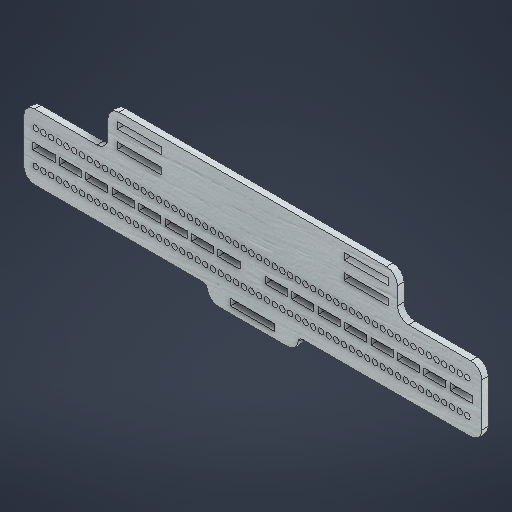
# Autodesk Inventor part: side_frame
Saved by Autodesk Inventor 2025.3 (Build 293356030, 356C)
## iProperties
Created: 2025-09-04
Part Number: side_frame
Material: 木材 (楓木)
Document SubType Name: Modeling
Designer: 陳泓任
Density: 0.67 g/cm^3
Appearance: 木材 - 白色刷漆
Author: 陳泓任
Autodesk Inventor part; units mm, degrees
ref_plane "YZ Plane" through (0, 0, 0) normal (1, 0, 0) x (0, 1, 0)
ref_plane "XZ Plane" through (0, 0, 0) normal (0, 1, 0) x (-1, 0, 0)
ref_plane "XY Plane" through (0, 0, 0) normal (0, 0, 1) x (1, 0, 0)
sketch "草圖1" plane through (0, 0, 0) normal (0, 0, 1) x (1, 0, 0)
  line L0 (41.49, 17.7685) -> (41.49, 20.7685)
  line L1 (41.49, 20.7685) -> (61.49, 20.7685)
  line L2 (61.49, 20.7685) -> (61.49, 17.7685)
  line L3 (61.49, 17.7685) -> (41.49, 17.7685)
  arc A0 (99, -14.8985) -> (104, -9.8985) centre (99, -9.8985) ccw
  arc A1 (-104, -9.8985) -> (-99, -14.8985) centre (-99, -9.8985) ccw
  line L4 (-61.49, 17.7685) -> (-61.49, 20.7685)
  line L5 (-61.49, 20.7685) -> (-41.49, 20.7685)
  line L6 (-41.49, 20.7685) -> (-41.49, 17.7685)
  line L7 (-41.49, 17.7685) -> (-61.49, 17.7685)
  arc A2 (65.74, 27.7685) -> (60.74, 32.7685) centre (60.74, 27.7685) ccw
  circle A3 centre (-98.5092, 7.5) radius 1.25
  circle A4 centre (-98.5092, -7.5) radius 1.25
  arc A5 (-70.74, 14.8985) -> (-65.74, 19.8985) centre (-70.74, 19.8985) ccw
  arc A6 (104, 9.8985) -> (99, 14.8985) centre (99, 9.8985) ccw
  arc A7 (-99, 14.8985) -> (-104, 9.8985) centre (-99, 9.8985) ccw
  arc A8 (65.74, 19.8985) -> (70.74, 14.8985) centre (70.74, 19.8985) ccw
  line L8 (-99, -14.8985) -> (-22.615, -14.8985)
  arc A9 (15.6624, -21.0852) -> (20.6286, -16.6661) centre (15.6624, -16.0852) ccw
  arc A10 (22.615, -14.8985) -> (20.6286, -16.6661) centre (22.615, -16.8985) ccw
  line L9 (-10, -18.0852) -> (-10, -15.0852)
  line L10 (-10, -15.0852) -> (10, -15.0852)
  line L11 (10, -15.0852) -> (10, -18.0852)
  line L12 (10, -18.0852) -> (-10, -18.0852)
  arc A11 (-20.6286, -16.6661) -> (-22.615, -14.8985) centre (-22.615, -16.8985) ccw
  arc A12 (-20.6286, -16.6661) -> (-15.6624, -21.0852) centre (-15.6624, -16.0852) ccw
  line L13 (-65.74, 27.7685) -> (-65.74, 19.8985)
  line L14 (-104, 9.8985) -> (-104, -9.8985)
  line L15 (104, 9.8985) -> (104, -9.8985)
  line L16 (-15.6624, -21.0852) -> (15.6624, -21.0852)
  line L17 (22.615, -14.8985) -> (99, -14.8985)
  line L18 (70.74, 14.8985) -> (99, 14.8985)
  line L19 (-99, 14.8985) -> (-70.74, 14.8985)
  line L20 (0, -35.3826) -> (0, 51.5191)
  line L21 (-104.9871, 0) -> (119.3176, 0)
  circle A13 centre (-95.0092, 7.5) radius 1.25
  circle A14 centre (-95.0092, -7.5) radius 1.25
  circle A15 centre (-91.5092, 7.5) radius 1.25
  circle A16 centre (-91.5092, -7.5) radius 1.25
  circle A17 centre (-88.0092, 7.5) radius 1.25
  circle A18 centre (-88.0092, -7.5) radius 1.25
  circle A19 centre (-84.5092, 7.5) radius 1.25
  circle A20 centre (-84.5092, -7.5) radius 1.25
  circle A21 centre (-81.0092, 7.5) radius 1.25
  circle A22 centre (-81.0092, -7.5) radius 1.25
  circle A23 centre (-77.5092, 7.5) radius 1.25
  circle A24 centre (-77.5092, -7.5) radius 1.25
  circle A25 centre (-74.0092, 7.5) radius 1.25
  circle A26 centre (-74.0092, -7.5) radius 1.25
  circle A27 centre (-70.5092, 7.5) radius 1.25
  circle A28 centre (-70.5092, -7.5) radius 1.25
  circle A29 centre (-67.0092, 7.5) radius 1.25
  circle A30 centre (-67.0092, -7.5) radius 1.25
  circle A31 centre (-63.5092, 7.5) radius 1.25
  circle A32 centre (-63.5092, -7.5) radius 1.25
  circle A33 centre (-60.0092, 7.5) radius 1.25
  circle A34 centre (-60.0092, -7.5) radius 1.25
  circle A35 centre (-56.5092, 7.5) radius 1.25
  circle A36 centre (-56.5092, -7.5) radius 1.25
  circle A37 centre (-53.0092, 7.5) radius 1.25
  circle A38 centre (-53.0092, -7.5) radius 1.25
  circle A39 centre (-49.5092, 7.5) radius 1.25
  circle A40 centre (-49.5092, -7.5) radius 1.25
  circle A41 centre (-46.0092, 7.5) radius 1.25
  circle A42 centre (-46.0092, -7.5) radius 1.25
  circle A43 centre (-42.5092, 7.5) radius 1.25
  circle A44 centre (-42.5092, -7.5) radius 1.25
  circle A45 centre (-39.0092, 7.5) radius 1.25
  circle A46 centre (-39.0092, -7.5) radius 1.25
  circle A47 centre (-35.5092, 7.5) radius 1.25
  circle A48 centre (-35.5092, -7.5) radius 1.25
  circle A49 centre (-32.0092, 7.5) radius 1.25
  circle A50 centre (-32.0092, -7.5) radius 1.25
  circle A51 centre (-28.5092, 7.5) radius 1.25
  circle A52 centre (-28.5092, -7.5) radius 1.25
  circle A53 centre (-25.0092, 7.5) radius 1.25
  circle A54 centre (-25.0092, -7.5) radius 1.25
  circle A55 centre (-21.5092, 7.5) radius 1.25
  circle A56 centre (-21.5092, -7.5) radius 1.25
  circle A57 centre (-18.0092, 7.5) radius 1.25
  circle A58 centre (-18.0092, -7.5) radius 1.25
  circle A59 centre (-14.5092, 7.5) radius 1.25
  circle A60 centre (-14.5092, -7.5) radius 1.25
  circle A61 centre (-11.0092, 7.5) radius 1.25
  circle A62 centre (-11.0092, -7.5) radius 1.25
  circle A63 centre (-7.5092, 7.5) radius 1.25
  circle A64 centre (-7.5092, -7.5) radius 1.25
  circle A65 centre (-4.0092, 7.5) radius 1.25
  circle A66 centre (-4.0092, -7.5) radius 1.25
  circle A67 centre (-0.5092, 7.5) radius 1.25
  circle A68 centre (-0.5092, -7.5) radius 1.25
  circle A69 centre (2.9908, 7.5) radius 1.25
  circle A70 centre (2.9908, -7.5) radius 1.25
  circle A71 centre (6.4908, 7.5) radius 1.25
  circle A72 centre (6.4908, -7.5) radius 1.25
  circle A73 centre (9.9908, 7.5) radius 1.25
  circle A74 centre (9.9908, -7.5) radius 1.25
  circle A75 centre (13.4908, 7.5) radius 1.25
  circle A76 centre (13.4908, -7.5) radius 1.25
  circle A77 centre (16.9908, 7.5) radius 1.25
  circle A78 centre (16.9908, -7.5) radius 1.25
  circle A79 centre (20.4908, 7.5) radius 1.25
  circle A80 centre (20.4908, -7.5) radius 1.25
  circle A81 centre (23.9908, 7.5) radius 1.25
  circle A82 centre (23.9908, -7.5) radius 1.25
  circle A83 centre (27.4908, 7.5) radius 1.25
  circle A84 centre (27.4908, -7.5) radius 1.25
  circle A85 centre (30.9908, 7.5) radius 1.25
  circle A86 centre (30.9908, -7.5) radius 1.25
  circle A87 centre (34.4908, 7.5) radius 1.25
  circle A88 centre (34.4908, -7.5) radius 1.25
  circle A89 centre (37.9908, 7.5) radius 1.25
  circle A90 centre (37.9908, -7.5) radius 1.25
  circle A91 centre (41.4908, 7.5) radius 1.25
  circle A92 centre (41.4908, -7.5) radius 1.25
  circle A93 centre (44.9908, 7.5) radius 1.25
  circle A94 centre (44.9908, -7.5) radius 1.25
  circle A95 centre (48.4908, 7.5) radius 1.25
  circle A96 centre (48.4908, -7.5) radius 1.25
  circle A97 centre (51.9908, 7.5) radius 1.25
  circle A98 centre (51.9908, -7.5) radius 1.25
  circle A99 centre (55.4908, 7.5) radius 1.25
  circle A100 centre (55.4908, -7.5) radius 1.25
  circle A101 centre (58.9908, 7.5) radius 1.25
  circle A102 centre (58.9908, -7.5) radius 1.25
  circle A103 centre (62.4908, 7.5) radius 1.25
  circle A104 centre (62.4908, -7.5) radius 1.25
  circle A105 centre (65.9908, 7.5) radius 1.25
  circle A106 centre (65.9908, -7.5) radius 1.25
  circle A107 centre (69.4908, 7.5) radius 1.25
  circle A108 centre (69.4908, -7.5) radius 1.25
  circle A109 centre (72.9908, 7.5) radius 1.25
  circle A110 centre (72.9908, -7.5) radius 1.25
  circle A111 centre (76.4908, 7.5) radius 1.25
  circle A112 centre (76.4908, -7.5) radius 1.25
  circle A113 centre (79.9908, 7.5) radius 1.25
  circle A114 centre (79.9908, -7.5) radius 1.25
  circle A115 centre (83.4908, 7.5) radius 1.25
  circle A116 centre (83.4908, -7.5) radius 1.25
  circle A117 centre (86.9908, 7.5) radius 1.25
  circle A118 centre (86.9908, -7.5) radius 1.25
  circle A119 centre (90.4908, 7.5) radius 1.25
  circle A120 centre (90.4908, -7.5) radius 1.25
  circle A121 centre (93.9908, 7.5) radius 1.25
  circle A122 centre (93.9908, -7.5) radius 1.25
  circle A123 centre (97.4908, 7.5) radius 1.25
  circle A124 centre (97.4908, -7.5) radius 1.25
  line L22 (65.74, 27.7685) -> (65.74, 19.8985)
  line L23 (-98.5092, 7.5) -> (-98.5092, -7.5)
  line L24 (-60.74, 32.7685) -> (60.74, 32.7685)
  arc A125 (-60.74, 32.7685) -> (-65.74, 27.7685) centre (-60.74, 27.7685) ccw
  line L25 (-61.49, 28.7685) -> (-41.49, 28.7685)
  line L26 (-61.49, 25.7685) -> (-61.49, 28.7685)
  line L27 (-41.49, 25.7685) -> (-61.49, 25.7685)
  line L28 (-41.49, 28.7685) -> (-41.49, 25.7685)
  line L29 (41.49, 28.7685) -> (61.49, 28.7685)
  line L30 (41.49, 25.7685) -> (41.49, 28.7685)
  line L31 (61.49, 25.7685) -> (41.49, 25.7685)
  line L32 (61.49, 28.7685) -> (61.49, 25.7685)
  point P0 (0, 0)
  point P1 (-65.74, 32.7685)
  point P2 (0, -15.0852)
  point P3 (-104, 0)
  point P4 (0, 32.7638)
  dimension "d0" = 20
  dimension "d1" = 3
  dimension "d2" = 3
  dimension "d4" = 2.5
  dimension "d7" = 4.25
  dimension "d11" = 5
  dimension "d12" = 2
  dimension "d14" = 5.4908
  dimension "d16" = 15
  dimension "d19" = 3.5
  dimension "d26" = 29.797
  dimension "d29" = 45.23
  dimension "d30" = 31.3249
  dimension "d43" = 208
  dimension "d44" = 4.25
  dimension "d45" = 5
  dimension "d46" = 17.87
  dimension "d48" = 38.26
  dimension "d49" = 12
  dimension "d54" = 8
  constraints: 126 centre point, 66 end point, 24 point on circle, 22 tangent, 10 equal radius, 7 point on line, 6 horizontal, 6 parallel, 5 perpendicular, 5 vertical, 4 collinear, 2 midpoint, 244 other
  measures "d0" distance of L11.end L9.start
  measures "d1" distance of L9.start L9.end
  measures "d2" distance between parallel lines of L16 L12
  measures "d4" diameter of A3
  measures "d7" distance between parallel lines of L13 L4
  measures "d11" radius of A2
  measures "d12" radius of A11
  measures "d14" distance from line of L14 L23.start
  measures "d16" distance of L23.end L23.start
  measures "d19" distance of L23.start A13.centre
  measures "d26" distance between parallel lines of L18 L17
  measures "d29" distance of A10.centre A11.centre
  measures "d30" distance of L16.start L16.end
  measures "d43" diameter of L14 L20
  measures "d44" distance between parallel lines of L22 L2
  measures "d45" radius of A125
  measures "d46" distance between parallel lines of L19 L24
  measures "d48" distance between parallel lines of L22 L15
  measures "d49" distance between parallel lines of L5 L24
  measures "d54" distance of L4.end L25.start
extrude "擠出1" add sketch "草圖1" along normal blind 3 contours L17 A10 A9 L16 L20 L12 L11 L10 A68 L21 L15 A0 | L21 L20 A67 L24 A2 L22 A8 L18 A6 L15 | L21 L14 A7 L19 A5 L13 A125 L24 L20 A67 | L20 A68 L10 L9 L12 L16 A12 A11 L8 A1 L14 L21
sketch "草圖2" plane through (0, 0, 3) normal (0, 0, 1) x (1, 0, 0)
  line L0 (-104.9871, 0) -> (119.3176, 0) projected
  line L1 (0, -35.3826) -> (0, 51.5191) projected
  line L2 (-99.7592, 1.5) -> (-89.7592, 1.5)
  line L3 (-89.7592, 1.5) -> (-89.7592, -1.5)
  line L4 (-89.7592, -1.5) -> (-99.7592, -1.5)
  line L5 (-99.7592, -1.5) -> (-99.7592, 1.5)
  circle A0 centre (-98.5092, 7.5) radius 1.25 projected
  circle A1 centre (-98.5092, -7.5) radius 1.25 projected
  line L6 (-87.7592, 1.5) -> (-77.7592, 1.5)
  line L7 (-77.7592, -1.5) -> (-87.7592, -1.5)
  line L8 (-87.7592, -1.5) -> (-87.7592, 1.5)
  line L9 (-77.7592, 1.5) -> (-77.7592, -1.5)
  line L10 (-75.7592, 1.5) -> (-65.7592, 1.5)
  line L11 (-65.7592, -1.5) -> (-75.7592, -1.5)
  line L12 (-75.7592, -1.5) -> (-75.7592, 1.5)
  line L13 (-65.7592, 1.5) -> (-65.7592, -1.5)
  line L14 (-63.7592, 1.5) -> (-53.7592, 1.5)
  line L15 (-53.7592, -1.5) -> (-63.7592, -1.5)
  line L16 (-63.7592, -1.5) -> (-63.7592, 1.5)
  line L17 (-53.7592, 1.5) -> (-53.7592, -1.5)
  line L18 (-51.7592, 1.5) -> (-41.7592, 1.5)
  line L19 (-41.7592, -1.5) -> (-51.7592, -1.5)
  line L20 (-51.7592, -1.5) -> (-51.7592, 1.5)
  line L21 (-41.7592, 1.5) -> (-41.7592, -1.5)
  line L22 (-39.7592, 1.5) -> (-29.7592, 1.5)
  line L23 (-29.7592, -1.5) -> (-39.7592, -1.5)
  line L24 (-39.7592, -1.5) -> (-39.7592, 1.5)
  line L25 (-29.7592, 1.5) -> (-29.7592, -1.5)
  line L26 (-27.7592, 1.5) -> (-17.7592, 1.5)
  line L27 (-17.7592, -1.5) -> (-27.7592, -1.5)
  line L28 (-27.7592, -1.5) -> (-27.7592, 1.5)
  line L29 (-17.7592, 1.5) -> (-17.7592, -1.5)
  line L30 (-15.7592, 1.5) -> (-5.7592, 1.5)
  line L31 (-5.7592, -1.5) -> (-15.7592, -1.5)
  line L32 (-15.7592, -1.5) -> (-15.7592, 1.5)
  line L33 (-5.7592, 1.5) -> (-5.7592, -1.5)
  line L34 (99.7592, 1.5) -> (89.7592, 1.5)
  line L35 (89.7592, 1.5) -> (89.7592, -1.5)
  line L36 (89.7592, -1.5) -> (99.7592, -1.5)
  line L37 (99.7592, -1.5) -> (99.7592, 1.5)
  line L38 (87.7592, 1.5) -> (77.7592, 1.5)
  line L39 (77.7592, -1.5) -> (87.7592, -1.5)
  line L40 (87.7592, -1.5) -> (87.7592, 1.5)
  line L41 (77.7592, 1.5) -> (77.7592, -1.5)
  line L42 (75.7592, 1.5) -> (65.7592, 1.5)
  line L43 (65.7592, -1.5) -> (75.7592, -1.5)
  line L44 (75.7592, -1.5) -> (75.7592, 1.5)
  line L45 (65.7592, 1.5) -> (65.7592, -1.5)
  line L46 (63.7592, 1.5) -> (53.7592, 1.5)
  line L47 (53.7592, -1.5) -> (63.7592, -1.5)
  line L48 (63.7592, -1.5) -> (63.7592, 1.5)
  line L49 (53.7592, 1.5) -> (53.7592, -1.5)
  line L50 (51.7592, 1.5) -> (41.7592, 1.5)
  line L51 (41.7592, -1.5) -> (51.7592, -1.5)
  line L52 (51.7592, -1.5) -> (51.7592, 1.5)
  line L53 (41.7592, 1.5) -> (41.7592, -1.5)
  line L54 (39.7592, 1.5) -> (29.7592, 1.5)
  line L55 (29.7592, -1.5) -> (39.7592, -1.5)
  line L56 (39.7592, -1.5) -> (39.7592, 1.5)
  line L57 (29.7592, 1.5) -> (29.7592, -1.5)
  line L58 (27.7592, 1.5) -> (17.7592, 1.5)
  line L59 (17.7592, -1.5) -> (27.7592, -1.5)
  line L60 (27.7592, -1.5) -> (27.7592, 1.5)
  line L61 (17.7592, 1.5) -> (17.7592, -1.5)
  line L62 (15.7592, 1.5) -> (5.7592, 1.5)
  line L63 (5.7592, -1.5) -> (15.7592, -1.5)
  line L64 (15.7592, -1.5) -> (15.7592, 1.5)
  line L65 (5.7592, 1.5) -> (5.7592, -1.5)
  point P0 (0, 0)
  point P1 (-99.7592, 0)
  point P2 (-87.7592, 0)
  point P3 (-75.7592, 0)
  point P4 (-63.7592, 0)
  point P5 (-51.7592, 0)
  point P6 (-39.7592, 0)
  point P7 (-27.7592, 0)
  point P8 (-15.7592, 0)
  point P9 (99.7592, 0)
  point P10 (87.7592, 0)
  point P11 (75.7592, 0)
  point P12 (63.7592, 0)
  point P13 (51.7592, 0)
  point P14 (39.7592, 0)
  point P15 (27.7592, 0)
  point P16 (15.7592, 0)
  point P17 (15.7592, 0)
  point P18 (5.7592, 0)
  dimension "d33" = 3
  dimension "d34" = 10
  dimension "d38" = 12
  constraints: 128 end point, 40 symmetric about line, 2 horizontal, 2 parallel, 1 midpoint, 1 perpendicular, 1 tangent, 64 other
  measures "d33" distance of L2.end L3.end
  measures "d34" distance of L3.end L4.end
  measures "d38" distance of L2.start L6.start
extrude "擠出2" cut sketch "草圖2" against normal up to surface (3 mm away) contours L5 L2 L3 L0 | L0 L3 L4 L5 | L35 L34 L37 L0 | L0 L37 L36 L35 | L41 L38 L40 L0 | L0 L40 L39 L41 | L45 L42 L44 L0 | L0 L44 L43 L45 | L49 L46 L48 L0 | L0 L48 L47 L49 | L53 L50 L52 L0 | L0 L52 L51 L53 | L57 L54 L56 L0 | L0 L56 L55 L57 | L61 L58 L60 L0 | L0 L60 L59 L61 | L65 L62 L64 L0 | L0 L64 L63 L65 | L32 L30 L33 L0 | L0 L33 L31 L32 | L28 L26 L29 L0 | L0 L29 L27 L28 | L24 L22 L25 L0 | L0 L25 L23 L24 | L20 L18 L21 L0 | L0 L21 L19 L20 | L16 L14 L17 L0 | L0 L17 L15 L16 | L12 L10 L13 L0 | L0 L13 L11 L12 | L8 L6 L9 L0 | L0 L9 L7 L8
sketch "草圖3" plane through (0, 0, 3) normal (0, 0, 1) x (1, 0, 0)
  line L0 (0, 52.3829) -> (0, -39.0235)
  line L1 (-112.5881, 0) -> (123.4866, 0)
  point P0 (0, 0)
  constraints: 4 end point, 2 point on line, 1 horizontal, 1 vertical
